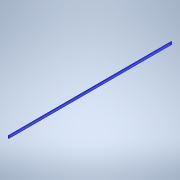
# Autodesk Inventor part: DR成形フレキラックDR1-2000KHK
Saved by Autodesk Inventor 2022 (Build 260153070, 153G)
## iProperties
Created: 2022-08-02
Part Number: DR成形フレキラックDR1-2000KHK
Material: ABS プラスチック
Document SubType Name: Modeling
Designer: zegi
Density: 1.06 g/cm^3
Appearance: 青 - 壁塗料 - 光沢
Author: zegi
Autodesk Inventor part; units mm, degrees
ref_plane "YZ Plane" through (0, 0, 0) normal (1, 0, 0) x (0, 1, 0)
ref_plane "XZ Plane" through (0, 0, 0) normal (0, 1, 0) x (-1, 0, 0)
ref_plane "XY Plane" through (0, 0, 0) normal (0, 0, 1) x (1, 0, 0)
sketch "スケッチ1" plane through (0, 0, 0) normal (0, 0, 1) x (1, 0, 0)
  line L0 (0, 0) -> (3.3, 0)
  line L1 (3.3, 0) -> (3.3, 10)
  line L2 (3.3, 10) -> (0, 10)
  line L3 (0, 10) -> (0, 0)
  dimension "d0" = 3.3
  dimension "d1" = 10
  constraints: 8 end point, 2 parallel, 1 horizontal, 1 perpendicular
  measures "d0" distance of L2.end L1.end
  measures "d1" distance of L1.end L0.end
extrude "押し出し1" add sketch "スケッチ1" along normal blind 710
sketch "スケッチ2" plane through (3.3, 10, 710) normal (1, 0, 0) x (0, 0, -1)
  line L0 (710, -10) -> (710, 0) projected
  line L1 (710, 0) -> (0, 0) projected
  line L2 (0, -10) -> (0, 0) projected
  point P0 (705, -5)
  point P1 (5, -5)
  dimension "d4" = 5
  dimension "d5" = 5
  dimension "d6" = 5
  dimension "d7" = 5
  measures "d4" distance from line of L0 point (705, -5)
  measures "d5" distance from line of L1 point (705, -5)
  measures "d6" distance from line of L2 point (5, -5)
  measures "d7" distance from line of L1 point (5, -5)
hole "穴1" at (3.3, 5, 5) at (3.3, 5, 705) direction (-1, 0, 0) diameter 3 end through all
